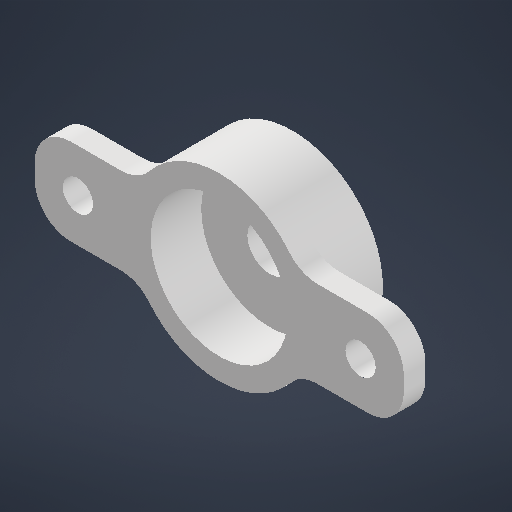
# Autodesk Inventor part: для подшипника 25-26
Saved by Autodesk Inventor 2026.2 (Build 302298000, 298)
## iProperties
Created: 2025-11-08
Part Number: для подшипника 25-26
Material: Типовые
Document SubType Name: Modeling
Designer: Phantom
Density: 1 g/cm^3
Appearance: По умолчанию
Author: Phantom
Autodesk Inventor part; units mm, degrees
ref_plane "YZ Plane" through (0, 0, 0) normal (1, 0, 0) x (0, 1, 0)
ref_plane "XZ Plane" through (0, 0, 0) normal (0, 1, 0) x (-1, 0, 0)
ref_plane "XY Plane" through (0, 0, 0) normal (0, 0, 1) x (1, 0, 0)
sketch "Эскиз1" plane through (0, 0, 0) normal (0, 0, 1) x (1, 0, 0)
  circle A0 centre (0, 0) radius 9.5
  circle A1 centre (0, 0) radius 12.5
  circle A2 centre (0, 0) radius 19.6
  circle A3 centre (-19.6, 0) radius 2.1
  circle A4 centre (19.6, 0) radius 2.1
  line L0 (-21.7, 0) -> (21.7, 0)
  line L1 (-25.6, 6) -> (25.6, 6)
  line L2 (-25.6, -6) -> (25.6, -6)
  line L3 (-25.6, 6) -> (-25.6, -6)
  line L4 (0, 0) -> (0, 6)
  line L5 (25.6, 6) -> (25.6, -6)
  point P0 (10.9659, -6)
  point P1 (10.9659, 6)
  point P2 (-10.9659, 6)
  point P3 (-10.9659, -6)
  dimension "d3" = 4.2
  dimension "d4" = 4.2
  dimension "d0" = 19
  dimension "d1" = 25
  dimension "d2" = 39.2
  dimension "d5" = 6
  dimension "d6" = 6
  dimension "d7" = 6
  constraints: 12 end point, 3 centre point, 3 coincident, 2 horizontal alignment, 2 parallel, 2 point on circle, 2 symmetric about line, 1 horizontal, 1 midpoint, 1 perpendicular, 1 vertical, 4 other
  measures "d0" diameter of A0
  measures "d1" diameter of A1
  measures "d2" diameter of A2
  measures "d5" distance between parallel lines of L0 L1
  measures "d6" distance between parallel lines of L0 L2
  measures "d7" distance from line of A2.start L3
extrude "Выдавливание1" add sketch "Эскиз1" along normal blind 3 contours L0 A1 L2 A0 | A0 L1 A1 L0 | A0 L1 A1 | L2 A1 A0 | L0 A4 A2 L2 A1 | A1 L1 A2 A4 L0 | A0 L0 A1 L1 | L2 A1 L0 A0 | A1 L0 A3 A2 L1 | L1 L5 L2 A2 A4 | L2 A2 A3 L0 A1 | A2 A3 L2 L3 L1
sketch "Эскиз2" plane through (0, 0, 0) normal (0, 0, -1) x (-1, 0, 0)
  line L0 (-25.6, -6) -> (-25.6, 6) projected
  line L1 (-10.9659, -6) -> (-25.6, -6) projected
  arc A0 (-10.9659, -6) -> (10.9659, -6) centre (0, 0) ccw projected
  line L2 (25.6, -6) -> (10.9659, -6) projected
  line L3 (25.6, 6) -> (25.6, -6) projected
  line L4 (10.9659, 6) -> (25.6, 6) projected
  arc A1 (10.9659, 6) -> (-10.9659, 6) centre (0, 0) ccw projected
  line L5 (-25.6, 6) -> (-10.9659, 6) projected
  circle A2 centre (-19.6, 0) radius 2.1 projected
  circle A3 centre (19.6, 0) radius 2.1 projected
  circle A4 centre (0, 0) radius 9.5 projected
  circle A5 centre (0, 0) radius 12.5
  point P0 (-10.9659, 6)
  constraints: 1 centre point, 1 coincident, 1 concentric
extrude "Выдавливание2" add sketch "Эскиз2" along normal blind 4 contours A5 A1 A0
sketch "Эскиз3" plane through (0, 0, -4) normal (0, 0, -1) x (-1, 0, 0)
  circle A0 centre (0, 0) radius 12.5 projected
  circle A1 centre (0, 0) radius 9.5 projected
  circle A2 centre (0, 0) radius 3.1
  dimension "d12" = 6.2
  constraints: 1 centre point, 1 coincident
  measures "d12" diameter of A2
extrude "Выдавливание3" add sketch "Эскиз3" along normal blind 3.2 contours A0 | A1
fillet "Сопряжение1" radius 5 8 edges at (-25.6, 6, 1.5) (-25.6, -6, 1.5) (25.6, 6, 1.5) (25.6, -6, 1.5) (10.9659, -6, 1.5) (10.9659, 6, 1.5) (-10.9659, 6, 1.5) (-10.9659, -6, 1.5)
